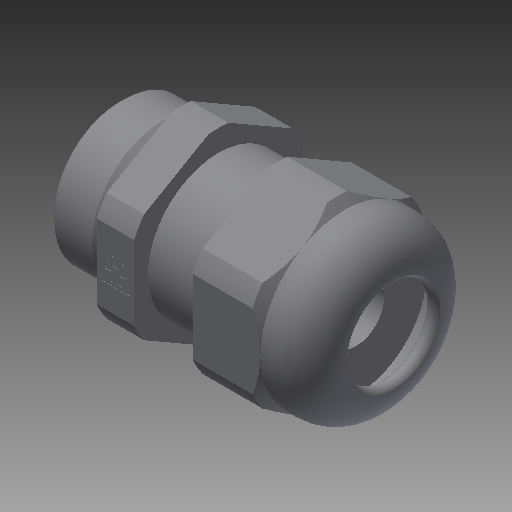
# Autodesk Inventor part: SKINTOP ST PG 16      Art. Nr. 53015240(F=9) Kunststoff
Saved by Autodesk Inventor 2019.3 (Build 233278000, 278)
## iProperties
Category: PARTsolutions
Company: LAPP
Created: 2018-12-14
Part Number: SKINTOP ST PG 16      Art. Nr. 53015240(F=9) Kunststoff
Material: Generic
Catalog Web Link: www.cadenas.de
Description: SKINTOP® ST-Cable gland plastic
Vendor: LAPP
Document SubType Name: Modeling
Designer: psadmin
Manufacturer: LAPP
Mass: 17.8396 g
Surface Area: 66.507 cm^2
Volume: 17.8396 cm^3
Density: 1 g/cm^3
Appearance: PSOLRGB-175-175-175
PSOL_IDENT_0: {$CADENAS_DATA\23d-libs\lapp_kabel\skintop_kabelverschraubungen\skintop_kabelverschraubungen_polyami
PSOL_IDENT_1: d_pg\skintop_kabelverschraubungen_polyamid_pg\st_pg.prj},231 {VTYP=3D},{NB=SKINTOP ST PG 16      Art
PSOL_IDENT_2: . Nr. 53015240(F=9)},{LINA=SKINTOP ST PG 16      Art. Nr. 53015240},{NN=SKINTOP® ST},{DATE=06.12.201
PSOL_IDENT_3: 8 13:21:11},{GEOMDATE=18.12.2013 09:14:44},{VERSION=},{LINEID=150},{WBVAR=F},{WBNUMERIC=F}  {NB=SKIN
PSOL_IDENT_4: TOP ST PG 16      Art. Nr. 53015240(F=9)},{LINA=SKINTOP ST PG 16      Art. Nr. 53015240},{KT=DUMMY},
PSOL_IDENT_5: {IDNR=},{ATN=53015240},{PG=PG 16},{ID=0.000},{RS=0.000},{FMIN=9.0},{FMAX=14.0},{F=9},{NDM=22.5},{X=9
PSOL_IDENT_6: .4},{SW=27},{A=29.5},{C=44.0},{D=10.0},{E=18.6},{H=10.8},{J=6.0},{K=6.0},{L=22.6},{XMAX=9.4},{RAL700
PSOL_IDENT_7: 1=},{RAL7035=},{RAL9005=X},{MATERIAL=Kunststoff},{VPE=MIN}
NN: SKINTOP® ST
NT: Cable gland plastic
NB: SKINTOP® ST PG 16      Art. Nr. 53015240(F=9)
NBSYN: SKINTOP® ST $PG.      Art. Nr. $ATN.(F=$F.)
LINA: SKINTOP® ST PG 16      Art. Nr. 53015240
ATN: 53015240
PG: PG 16
FMIN: 9
FMAX: 14
F: 9
SW: 27
A: 29.5
C: 44
D: 10
RAL9005: X
MATERIAL: Plastic
VPE: 0
SUPPLIER: LAPP
ARTICLENO: SKINTOP ST PG 16      Art. Nr. 53015240(F=9)
BOMINFO: SKINTOP ST PG 16      Art. Nr. 53015240
CREATOR: CADENAS GmbH
Title: SKINTOP ST PG 16      Art. Nr. 53015240
Author: Cadenas PARTsolutions
Comments: Cable gland plastic
Autodesk Inventor part; units mm, degrees
ref_plane "YZ Plane" through (0, 0, 0) normal (1, 0, 0) x (0, 1, 0)
ref_plane "XZ Plane" through (0, 0, 0) normal (0, 1, 0) x (-1, 0, 0)
ref_plane "XY Plane" through (0, 0, 0) normal (0, 0, 1) x (1, 0, 0)
sketch "Sketch_1" plane through (0, 0, 0) normal (0, 0, 1) x (1, 0, 0)
  line L0 (44, 0) -> (0, 0)
  line L1 (0, 10.0125) -> (0, 5.175)
  arc A0 (0, 5.175) -> (0.675, 4.5) centre (0.675, 5.175) ccw
  line L2 (0.675, 4.5) -> (38, 4.5)
  line L3 (38, 4.5) -> (38, 11.3)
  arc A1 (41.7763, 7.9237) -> (38, 11.3) centre (38, 7.5) ccw
  arc A2 (41.7763, 7.9237) -> (44, 7.5) centre (42.9628, 8.1034) ccw
  arc A3 (44, 7.5) -> (38, 13.5) centre (38, 7.5) ccw
  line L4 (38, 13.5) -> (36.2, 13.5)
  line L5 (36.2, 13.5) -> (31.7, 18)
  line L6 (31.7, 18) -> (25.4, 18)
  line L7 (25.4, 18) -> (25.4, 11.3)
  line L8 (25.4, 11.3) -> (16, 11.3)
  line L9 (16, 11.3) -> (16, 18)
  line L10 (16, 18) -> (10, 18)
  line L11 (10, 18) -> (10, 10.6875)
  line L12 (10, 10.6875) -> (8, 10.6875)
  line L13 (8, 10.6875) -> (7.0257, 11.25)
  line L14 (7.0257, 11.25) -> (1, 11.25)
  line L15 (1, 11.25) -> (1, 10.6875)
  line L16 (1, 10.6875) -> (0.675, 10.6875)
  arc A4 (0.675, 10.6875) -> (0, 10.0125) centre (0.675, 10.0125) ccw
  constraints: 34 end point, 10 point on circle, 5 centre point
revolve "Revolution1" add sketch "Sketch_1" angle 360 about axis through (44, 0, 0) along (-1, 0, 0)
sketch "Sketch_2" plane through (10, 0, 0) normal (1, 0, 0) x (0, 0, -1)
  line L0 (-27, 27) -> (-27, -27)
  line L1 (-27, -27) -> (27, -27)
  line L2 (27, -27) -> (27, 27)
  line L3 (27, 27) -> (-27, 27)
  arc A0 (-13.5, -5.9424) -> (-11.8963, -8.7201) centre (0, 0) ccw
  line L4 (-11.8963, -8.7201) -> (-1.6037, -14.6626)
  arc A1 (-1.6037, -14.6626) -> (1.6037, -14.6626) centre (0, 0) ccw
  line L5 (1.6037, -14.6626) -> (11.8963, -8.7201)
  arc A2 (11.8963, -8.7201) -> (13.5, -5.9424) centre (0, 0) ccw
  line L6 (13.5, -5.9424) -> (13.5, 5.9424)
  arc A3 (13.5, 5.9424) -> (11.8963, 8.7201) centre (0, 0) ccw
  line L7 (11.8963, 8.7201) -> (1.6037, 14.6626)
  arc A4 (1.6037, 14.6626) -> (-1.6037, 14.6626) centre (0, 0) ccw
  line L8 (-1.6037, 14.6626) -> (-11.8963, 8.7201)
  arc A5 (-11.8963, 8.7201) -> (-13.5, 5.9424) centre (0, 0) ccw
  line L9 (-13.5, 5.9424) -> (-13.5, -5.9424)
  constraints: 20 end point, 12 point on circle, 6 centre point
extrude "Extrusion1" cut sketch "Sketch_2" along normal blind 44
sketch "Skizze_1" plane through (0, 0, 13.5) normal (0, 0, 1) x (1, 0, 0)
  line L0 (10.8, 2.2) -> (10.8, -2.2)
  line L1 (10.8, -2.2) -> (15.2, -2.2)
  line L2 (15.2, -2.2) -> (15.2, 2.2)
  line L3 (15.2, 2.2) -> (10.8, 2.2)
  arc A0 (11.0456, 0.4247) -> (11.6685, -1.4924) centre (13, 0) ccw
  line L4 (11.6685, -1.4924) -> (11.759, -1.3678)
  arc A1 (12.0827, -1.6029) -> (11.759, -1.3678) centre (12.2947, -0.9708) ccw
  line L5 (12.0827, -1.6029) -> (11.9921, -1.7275)
  arc A2 (11.9921, -1.7275) -> (14.0079, -1.7275) centre (13, 0) ccw
  line L6 (14.0079, -1.7275) -> (13.9173, -1.6029)
  arc A3 (14.241, -1.3678) -> (13.9173, -1.6029) centre (13.7053, -0.9708) ccw
  line L7 (14.241, -1.3678) -> (14.3315, -1.4924)
  arc A4 (14.3315, -1.4924) -> (14.9544, 0.4247) centre (13, 0) ccw
  line L8 (14.9544, 0.4247) -> (14.8079, 0.3771)
  arc A5 (14.6843, 0.7576) -> (14.8079, 0.3771) centre (14.1413, 0.3708) ccw
  line L9 (14.6843, 0.7576) -> (14.8308, 0.8051)
  arc A6 (14.8308, 0.8051) -> (13.2, 1.99) centre (13, 0) ccw
  line L10 (13.2, 1.99) -> (13.2, 1.836)
  arc A7 (12.8, 1.836) -> (13.2, 1.836) centre (13, 1.2) ccw
  line L11 (12.8, 1.836) -> (12.8, 1.99)
  arc A8 (12.8, 1.99) -> (11.1692, 0.8051) centre (13, 0) ccw
  line L12 (11.1692, 0.8051) -> (11.3157, 0.7576)
  arc A9 (11.1921, 0.3771) -> (11.3157, 0.7576) centre (11.8587, 0.3708) ccw
  line L13 (11.1921, 0.3771) -> (11.0456, 0.4247)
  constraints: 28 end point, 20 point on circle, 10 centre point
extrude "Extrusion2" cut sketch "Skizze_1" against normal blind 0.054
body "Solid1"
